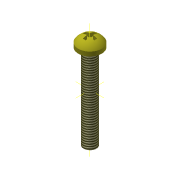
# Autodesk Inventor part: empty
Saved by Autodesk Inventor 2014 (Build 180170000, 170)
## iProperties
Created: 2015-04-13
Part Number: empty
Material: Generic
Document SubType Name: Modeling
Designer: Martin
Density: 1 g/cm^3
Appearance: Default
Author: Martin
Autodesk Inventor part; units mm, degrees
ref_plane "YZ Plane" through (0, 0, 0) normal (1, 0, 0) x (0, 1, 0)
ref_plane "XZ Plane" through (0, 0, 0) normal (0, 1, 0) x (-1, 0, 0)
sketch "Sketch1" plane through (0, 0, 0) normal (0, 1, 0) x (-1, 0, 0)
  line L0 (0, -15.8201) -> (0, 16.1707) projected
  line L1 (0, -11.25) -> (0, 11.25)
  line L2 (0, -11.25) -> (1.5, -11.25)
  line L3 (1.5, -11.25) -> (1.5, 8.75)
  line L4 (1.5, 8.75) -> (2.75, 8.75)
  line L5 (2.75, 8.75) -> (2.75, 9.75)
  arc A0 (2.75, 9.75) -> (0, 11.25) centre (0, 7.9792) ccw
  line L6 (3.5295, 0) -> (-0.5882, 0) projected
  point P0 (0, 0)
  dimension "d0" = 20
  dimension "d1" = 3
  dimension "d2" = 2.5
  dimension "d3" = 5.5
  dimension "d4" = 1
  constraints: 10 end point, 4 perpendicular, 2 point on circle, 2 point on line, 1 centre point, 1 line through centre, 1 symmetric about line
  measures "d0" distance of L2.end L3.end
  measures "d1" diameter of L3 L0
  measures "d2" distance from line of L4 L1.end
  measures "d3" diameter of L5 L0
  measures "d4" distance of L4.end L5.end
revolve "Revolution1" add sketch "Sketch1" angle 360 about axis through (0, 0, -10) along (0, 0, 1)
ref_plane "Work Plane1" through (0, 0, 11.25) normal (0, 0, 1) x (1, 0, 0)
sketch "Sketch2" plane through (0, 0, 11.25) normal (0, 0, 1) x (1, 0, 0)
  line L0 (-1.35, -0.35) -> (1.35, -0.35)
  line L1 (1.35, -0.35) -> (1.35, 0.35)
  line L2 (1.35, 0.35) -> (-1.35, 0.35)
  line L3 (-1.35, 0.35) -> (-1.35, -0.35)
  line L4 (-1.35, -0.35) -> (1.35, 0.35) construction
  line L5 (1.35, -0.35) -> (-1.35, 0.35) construction
  line L6 (0.35, -1.35) -> (-0.35, -1.35)
  line L7 (-0.35, -1.35) -> (-0.35, 1.35)
  line L8 (-0.35, 1.35) -> (0.35, 1.35)
  line L9 (0.35, 1.35) -> (0.35, -1.35)
  line L10 (0.35, -1.35) -> (-0.35, 1.35) construction
  line L11 (-0.35, -1.35) -> (0.35, 1.35) construction
  point P0 (0, 0)
  dimension "d6" = 2.7
  dimension "d7" = 0.7
  constraints: 24 end point, 4 midpoint, 4 parallel, 4 perpendicular, 2 horizontal
  measures "d6" distance of L8.end L6.start
  measures "d7" distance of L7.end L8.end
extrude "Extrusion1" cut sketch "Sketch2" against normal blind 1
thread "Thread1" size "M3x0.5" class "6g" standard "ANSI Metric M Profile" full length
body "Solid1"
